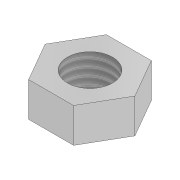
# Autodesk Inventor part: M4 nut
Saved by Autodesk Inventor 2020 (Build 240168000, 168)
## iProperties
Created: 2022-03-01
Part Number: M4 nut
Material: Generic
Document SubType Name: Modeling
Designer: ferrerx
Density: 1 g/cm^3
Appearance: Aluminum - Polished
Author: ferrerx
Autodesk Inventor part; units mm, degrees
ref_plane "YZ Plane" through (0, 0, 0) normal (1, 0, 0) x (0, 1, 0)
ref_plane "XZ Plane" through (0, 0, 0) normal (0, 1, 0) x (-1, 0, 0)
ref_plane "XY Plane" through (0, 0, 0) normal (0, 0, 1) x (1, 0, 0)
sketch "Sketch1" plane through (0, 0, 0) normal (0, 1, 0) x (-1, 0, 0)
  circle A0 centre (0, 0) radius 2
  line L0 (-1.9919, -3.45) -> (-3.9837, 0)
  line L1 (-3.9837, 0) -> (-1.9919, 3.45)
  line L2 (-1.9919, 3.45) -> (1.9919, 3.45)
  line L3 (1.9919, 3.45) -> (3.9837, 0)
  line L4 (3.9837, 0) -> (1.9919, -3.45)
  line L5 (1.9919, -3.45) -> (-1.9919, -3.45)
  line L6 (0, 0) -> (9.6963, 0) construction
  dimension "d0" = 6.9
  dimension "d1" = 4
  constraints: 14 end point, 2 coincident, 1 centre point, 1 horizontal, 1 parallel, 13 other
  measures "d0" distance between parallel lines of L2 L5
  measures "d1" diameter of A0
extrude "Extrusion1" add sketch "Sketch1" along normal blind 3.06
thread "Thread1" size "M4x0.7" class "6H" standard "ISO Metric profile" length 180
body "Solid1"
